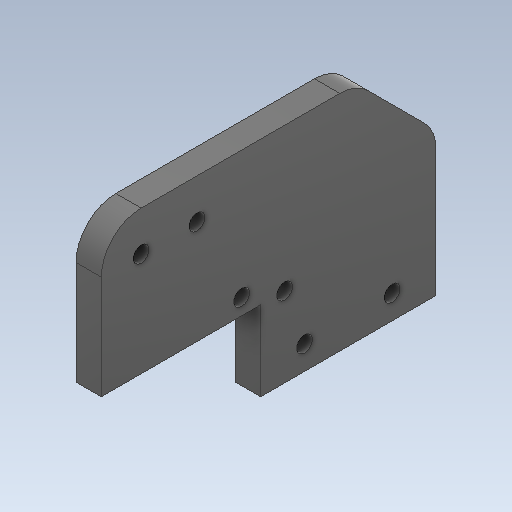
# Autodesk Inventor part: bodytoppart
Saved by Autodesk Inventor 2020.3 (Build 243373000, 373)
## iProperties
Created: 2021-06-21
Part Number: bodytoppart
Material: Steel, Mild
Document SubType Name: Modeling
Designer: 0x6f736f646f
Density: 7.85 g/cm^3
Appearance: Smooth - Black
Mass: 2806.13 g
Surface Area: 584.709 cm^2
Volume: 357.469 cm^3
Author: 0x6f736f646f
Autodesk Inventor part; units mm, degrees
ref_plane "YZ Plane" through (0, 0, 0) normal (1, 0, 0) x (0, 1, 0)
ref_plane "XZ Plane" through (0, 0, 0) normal (0, 1, 0) x (-1, 0, 0)
ref_plane "XY Plane" through (0, 0, 0) normal (0, 0, 1) x (1, 0, 0)
sketch "Sketch1" plane through (0, 0, 0) normal (1, 0, 0) x (0, 1, 0)
  line L0 (0, 0) -> (79.6447, 0)
  line L1 (140, 60.3553) -> (140, 185)
  line L2 (115, 210) -> (50, 210)
  line L3 (0, 110) -> (0, 0)
  arc A0 (140, 185) -> (115, 210) centre (115, 185) ccw
  line L4 (50, 210) -> (50, 110)
  line L5 (0, 110) -> (50, 110)
  circle A1 centre (115, 185) radius 5
  circle A2 centre (115, 150) radius 5
  circle A3 centre (60, 122) radius 5
  circle A4 centre (50, 95) radius 5
  line L6 (132.6777, 42.6777) -> (97.3223, 7.3223)
  arc A5 (132.6777, 42.6777) -> (140, 60.3553) centre (115, 60.3553) ccw
  arc A6 (79.6447, 0) -> (97.3223, 7.3223) centre (79.6447, 25) ccw
  circle A7 centre (15, 82.5) radius 5
  circle A8 centre (15, 27.5) radius 5
  point P0 (140, 210)
  point P1 (90, 0)
  dimension "d2" = 25
  dimension "d3" = 90
  dimension "d4" = 110
  dimension "d5" = 140
  dimension "d6" = 10
  dimension "d7" = 88
  dimension "d8" = 10
  dimension "d9" = 15
  dimension "d10" = 25
  dimension "d11" = 35
  dimension "d12" = 25
  dimension "d13" = 50
  dimension "d14" = 45
  dimension "d15" = 210
  dimension "d16" = 25
  dimension "d17" = 25
  dimension "d20" = 55
  dimension "d21" = 27.5
  dimension "d22" = 35
  dimension "d23" = 10
  constraints: 14 end point, 9 centre point, 6 point on circle, 6 tangent, 4 equal radius, 4 point on line, 3 vertical alignment, 2 horizontal, 2 parallel, 1 perpendicular, 1 vertical
  measures "d2" radius of A0
  measures "d3" distance between parallel lines of L4 L1
  measures "d4" distance between parallel lines of L0 L5
  measures "d5" distance between parallel lines of L3 L1
  measures "d6" diameter of A1
  measures "d7" distance from line of L2 A3.centre
  measures "d8" distance from line of L4 A3.centre
  measures "d9" distance from line of L5 A4.centre
  measures "d10" distance from line of L2 A1.centre
  measures "d11" distance of A2.centre A1.centre
  measures "d12" distance from line of A1.centre L1
  measures "d13" distance from line of point (90, 0) L1
  measures "d14" angle of L1 L6
  measures "d15" distance between parallel lines of L2 L0
  measures "d16" radius of A5
  measures "d17" radius of A6
  measures "d20" distance of A8.centre A7.centre
  measures "d21" distance from line of L0 A8.centre
  measures "d22" distance from line of A7.centre L4
  measures "d23" diameter of A8
extrude "Extrusion1" add sketch "Sketch1" along normal blind 15.875
body "Solid1"
